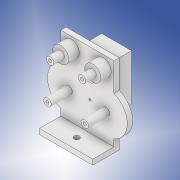
# Autodesk Inventor part: GA001
Saved by Autodesk Inventor 2017 SP1 (Build 210196100, 196)
## iProperties
Created: 2017-06-20
Part Number: GA001
Material: ABS Plastic
Document SubType Name: Modeling
Designer: zallen
Density: 1.06 g/cm^3
Appearance: CR White
Author: zallen
Autodesk Inventor part; units mm, degrees
ref_plane "YZ Plane" through (0, 0, 0) normal (1, 0, 0) x (0, 1, 0)
ref_plane "XZ Plane" through (0, 0, 0) normal (0, 1, 0) x (-1, 0, 0)
ref_plane "XY Plane" through (0, 0, 0) normal (0, 0, 1) x (1, 0, 0)
sketch "Sketch1" plane through (0, 0, 0) normal (0, 0, 1) x (1, 0, 0)
  line L0 (0, 0) -> (50, 0)
  line L1 (50, 0) -> (50, 75)
  line L2 (50, 75) -> (0, 75)
  line L3 (0, 75) -> (0, 0)
  dimension "d0" = 50
  dimension "d1" = 75
  constraints: 8 end point, 2 parallel, 1 horizontal, 1 perpendicular
  measures "d0" distance of L2.end L1.end
  measures "d1" distance of L1.end L0.end
extrude "Extrusion1" add sketch "Sketch1" along normal blind 5
sketch "Sketch2" plane through (0, 0, 0) normal (0, 1, 0) x (-1, 0, 0)
  line L0 (0, 5) -> (-50, 5) projected
  line L1 (0, 5) -> (-50, 5)
  line L2 (-50, 5) -> (-50, 25)
  line L3 (-50, 25) -> (0, 25)
  line L4 (0, 25) -> (0, 5)
  point P0 (0, 0)
  dimension "d4" = 20
  constraints: 8 end point, 2 parallel, 1 horizontal, 1 perpendicular, 1 vertical alignment
  measures "d4" distance of L1.end L2.end
extrude "Extrusion2" add sketch "Sketch2" along normal blind 5
sketch "Sketch3" plane through (0, 0, 5) normal (0, 0, 1) x (1, 0, 0)
  circle A0 centre (42.5, 30) radius 3.5
  circle A1 centre (40, 65) radius 3.5
  circle A2 centre (10, 65) radius 3.5
  circle A3 centre (7.5, 30) radius 3.5
  line L0 (42.5, 30) -> (7.5, 30) construction
  line L1 (50, 75) -> (0, 75) construction
  line L2 (25, 75) -> (25, 30) construction
  line L3 (10, 65) -> (40, 65) construction
  point P0 (0, 0)
  point P1 (25, 65)
  dimension "d7" = 7
  dimension "d8" = 7
  dimension "d9" = 7
  dimension "d10" = 7
  dimension "d12" = 30
  dimension "d14" = 10
  dimension "d30" = 35
  dimension "d32" = 35
  constraints: 6 end point, 4 centre point, 4 midpoint, 2 horizontal alignment, 1 coincident, 1 horizontal, 1 point on line, 1 vertical, 1 vertical alignment
  measures "d7" diameter of A0
  measures "d8" diameter of A1
  measures "d9" diameter of A2
  measures "d10" diameter of A3
  measures "d12" distance of L3.start L3.end
  measures "d14" vertical distance of point (25, 75) L3.end
  measures "d30" distance of L0.start L0.end
  measures "d32" distance between parallel lines of L0 L3
extrude "Extrusion3" add sketch "Sketch3" along normal blind 20
sketch "Sketch4" plane through (40, 65, 25) normal (0, 0, 1) x (1, 0, 0)
  circle A0 centre (-30, 0) radius 3.5 projected
  circle A1 centre (0, 0) radius 3.5 projected
  circle A2 centre (2.5, -35) radius 3.5 projected
  circle A3 centre (-32.5, -35) radius 3.5 projected
  circle A4 centre (-30, 0) radius 1.5
  circle A5 centre (0, 0) radius 1.5
  circle A6 centre (2.5, -35) radius 1.5
  circle A7 centre (-32.5, -35) radius 1.5
  point P0 (-40, -65)
  dimension "d17" = 3
  dimension "d18" = 3
  dimension "d19" = 3
  dimension "d20" = 3
  constraints: 4 centre point, 4 coincident
  measures "d17" diameter of A4
  measures "d18" diameter of A5
  measures "d19" diameter of A6
  measures "d20" diameter of A7
extrude "Extrusion4" cut sketch "Sketch4" against normal blind 10 contours A4 | A5 | A6 | A7
sketch "Sketch5" plane through (0, 5, 0) normal (0, 1, 0) x (1, 0, 0)
  circle A0 centre (25, -15) radius 2.5
  line L0 (0, -5) -> (50, -5) projected
  line L1 (0, -5) -> (0, -25) projected
  line L2 (0, -25) -> (50, -25) projected
  line L3 (50, -25) -> (50, -5) projected
  point P0 (0, 0)
  point P1 (0, -15)
  point P2 (25, -25)
  dimension "d23" = 5
  constraints: 2 midpoint, 1 centre point, 1 horizontal alignment, 1 vertical alignment
  measures "d23" diameter of A0
extrude "Extrusion5" cut sketch "Sketch5" against normal through all contours A0
sketch "Sketch6" plane through (0, 0, 5) normal (0, 0, 1) x (1, 0, 0)
  circle A0 centre (10, 65) radius 3.5 projected
  circle A1 centre (40, 65) radius 3.5 projected
  circle A2 centre (10, 65) radius 1.5 projected
  circle A3 centre (10, 65) radius 7.5
  circle A4 centre (40, 65) radius 7.5
  point P0 (0, 0)
  dimension "d26" = 15
  dimension "d27" = 15
  constraints: 2 centre point, 2 coincident
  measures "d26" diameter of A3
  measures "d27" diameter of A4
extrude "Extrusion6" add sketch "Sketch6" along normal blind 10 contours A3 | A4
sketch "Sketch8" plane through (0, 0, 0) normal (0, 0, -1) x (-1, 0, 0)
  circle A0 centre (-42.5, 30) radius 1.5 projected
  circle A1 centre (-42.5, 30) radius 20
  circle A2 centre (-7.5, 30) radius 3.5 projected
  circle A3 centre (-7.5, 30) radius 20
  point P0 (0, 0)
  dimension "d33" = 40
  dimension "d34" = 40
  constraints: 2 centre point, 2 coincident
  measures "d33" diameter of A1
  measures "d34" diameter of A3
extrude "Extrusion7" add sketch "Sketch8" against normal blind 5 contours A1 A3 | A1 A3 | A3 A1 | A2
sketch "Sketch9" plane through (0, 0, 5) normal (0, 0, 1) x (1, 0, 0)
  circle A0 centre (27.5, 50.5) radius 4.5
  line L0 (50, 75) -> (0, 75) projected
  line L1 (50, 75) -> (0, 75) construction
  line L2 (25, 75) -> (25, 35.564) construction
  point P0 (0, 0)
  dimension "d37" = 9
  dimension "d38" = 24.5
  dimension "d39" = 2.5
  constraints: 2 end point, 1 centre point, 1 midpoint, 1 vertical
  measures "d37" diameter of A0
  measures "d38" distance from line of L0 A0.centre
  measures "d39" distance from line of L2 A0.centre
extrude "Extrusion8" cut sketch "Sketch9" against normal through all
sketch "Sketch10" plane through (0, 0, 5) normal (0, 0, 1) x (1, 0, 0)
  circle A0 centre (27.5, 57.5) radius 1
  circle A1 centre (27.5, 32.1) radius 1
  line L0 (27.5, 57.5) -> (27.5, 32.1) construction
  circle A2 centre (27.5, 50.5) radius 4.5 projected
  point P0 (0, 0)
  dimension "d42" = 2
  dimension "d43" = 2
  dimension "d44" = 25.4
  dimension "d45" = 7
  constraints: 2 centre point, 2 end point, 1 vertical, 1 vertical alignment
  measures "d42" diameter of A0
  measures "d43" diameter of A1
  measures "d44" distance of L0.start L0.end
  measures "d45" distance of A2.centre L0.start
extrude "Extrusion9" cut sketch "Sketch10" against normal through all contours A0 | A1
sketch "Sketch11" plane through (0, 0, 0) normal (0, 0, -1) x (-1, 0, 0)
  circle A0 centre (-27.5, 57.5) radius 1 projected
  circle A1 centre (-27.5, 32.1) radius 1 projected
  circle A2 centre (-27.5, 57.5) radius 3
  circle A3 centre (-27.5, 32.1) radius 3
  point P0 (0, 0)
  dimension "d48" = 2
  dimension "d49" = 2
  constraints: 2 centre point
  measures "d48" radial gap between concentric circles of A0 A2
  measures "d49" radial gap between concentric circles of A1 A3
extrude "Extrusion10" add sketch "Sketch11" along normal blind 4
sketch "Sketch12" plane through (0, 0, 0) normal (0, 0, -1) x (-1, 0, 0)
  line L0 (-36.5, 28.1) -> (-18.5, 28.1)
  line L1 (-18.5, 28.1) -> (-18.5, 61.5)
  line L2 (-18.5, 61.5) -> (-36.5, 61.5)
  line L3 (-36.5, 61.5) -> (-36.5, 28.1)
  arc A0 (-28.815, 54.8036) -> (-26.185, 54.8036) centre (-27.5, 50.5) ccw projected
  line L4 (-50, 75) -> (0, 75) projected
  line L5 (-41.5, 23.1) -> (-13.5, 23.1)
  line L6 (-13.5, 23.1) -> (-13.5, 66.5)
  line L7 (-13.5, 66.5) -> (-41.5, 66.5)
  line L8 (-41.5, 66.5) -> (-41.5, 23.1)
  circle A1 centre (-27.5, 57.5) radius 1 projected
  circle A2 centre (-27.5, 32.1) radius 1 projected
  point P0 (0, 0)
  point P1 (-27.5, 61.5)
  dimension "d52" = 18
  dimension "d55" = 5
  dimension "d58" = 4
  dimension "d59" = 4
  constraints: 16 end point, 4 parallel, 2 perpendicular, 1 horizontal, 1 midpoint, 1 vertical alignment, 3 other
  measures "d52" distance of L0.start L0.end
  measures "d55" distance between parallel lines of L3 L8
  measures "d58" distance from line of A1.centre L2
  measures "d59" distance from line of L0 A2.centre
extrude "Extrusion11" add sketch "Sketch12" along normal blind 20 contours L8 L7 L6 L5
sketch "Sketch13" plane through (0, 0, -20) normal (0, 0, -1) x (-1, 0, 0)
  line L0 (-36.5, 28.1) -> (-36.5, 61.5) construction
  line L1 (-36.5, 61.5) -> (-18.5, 61.5) construction
  line L2 (-18.5, 61.5) -> (-18.5, 28.1) construction
  line L3 (-18.5, 28.1) -> (-36.5, 28.1) construction
  line L4 (-41.5, 23.1) -> (-13.5, 23.1) construction
  line L5 (-13.5, 23.1) -> (-13.5, 66.5) construction
  line L6 (-13.5, 66.5) -> (-41.5, 66.5) construction
  line L7 (-41.5, 66.5) -> (-41.5, 23.1) construction
  line L8 (-39, 64) -> (-16, 64) construction
  line L9 (-16, 64) -> (-16, 25.6) construction
  line L10 (-16, 25.6) -> (-39, 25.6) construction
  line L11 (-39, 25.6) -> (-39, 64) construction
  circle A0 centre (-39, 64) radius 1.5
  circle A1 centre (-16, 64) radius 1.5
  circle A2 centre (-16, 25.6) radius 1.5
  circle A3 centre (-39, 25.6) radius 1.5
  point P0 (0, 0)
  dimension "d60" = 2.5
  dimension "d61" = 3
  dimension "d62" = 3
  dimension "d63" = 3
  dimension "d64" = 3
  constraints: 8 end point, 4 centre point, 4 coincident, 3 other
  measures "d60" distance between parallel lines of L6 L8
  measures "d61" diameter of A0
  measures "d62" diameter of A1
  measures "d63" diameter of A2
  measures "d64" diameter of A3
extrude "Extrusion12" cut sketch "Sketch13" against normal blind 15
sketch "Sketch14" plane through (13.5, 23.1, 0) normal (0, -1, 0) x (1, 0, 0)
  line L0 (28, 0) -> (0, 0) projected
  line L1 (19, 0) -> (9, 0)
  line L2 (9, 0) -> (9, -10)
  line L3 (9, -10) -> (19, -10)
  line L4 (19, -10) -> (19, 0)
  line L5 (0, 0) -> (28, 0) projected
  point P0 (-13.5, 0)
  point P1 (14, 0)
  dimension "d67" = 10
  dimension "d68" = 10
  constraints: 8 end point, 3 midpoint, 2 parallel, 1 horizontal, 1 perpendicular, 1 point on line
  measures "d67" distance of L3.end L2.end
  measures "d68" distance of L2.end L1.end
extrude "Extrusion13" cut sketch "Sketch14" against normal blind 5
body "Solid1"
